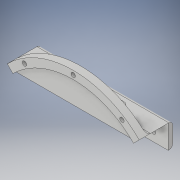
# Autodesk Inventor part: BearingGuard
Saved by Autodesk Inventor 2018 (Build 220112000, 112)
## iProperties
Created: 2019-02-07
Part Number: BearingGuard
Material: Generic
Document SubType Name: Modeling
Designer: anirudh
Density: 1 g/cm^3
Appearance: Default
Author: anirudh
Autodesk Inventor part; units mm, degrees
ref_plane "YZ Plane" through (0, 0, 0) normal (1, 0, 0) x (0, 1, 0)
ref_plane "XZ Plane" through (0, 0, 0) normal (0, 1, 0) x (-1, 0, 0)
ref_plane "XY Plane" through (0, 0, 0) normal (0, 0, 1) x (1, 0, 0)
sketch "Sketch1" plane through (0, 0, 0) normal (0, 0, 1) x (1, 0, 0)
  line L0 (0, 0) -> (101.6, 0)
  arc A0 (101.7181, 101.7181) -> (-0.1181, 101.7181) centre (50.8, 50.8) ccw
  arc A1 (106.4776, 106.4776) -> (-4.8776, 106.4776) centre (50.8, 50.8) ccw
  line L1 (0, 101.6) -> (-4.8776, 106.4776)
  line L2 (0, 101.6) -> (11.1798, 101.6) construction
  line L3 (101.6, 101.6) -> (106.4776, 106.4776)
  constraints: 8 end point, 4 point on circle, 2 centre point, 2 horizontal, 2 point on line, 1 coincident
extrude "Extrusion1" add sketch "Sketch1" along normal blind 2.54
sketch "Sketch2" plane through (0, 0, 0) normal (0, 0, -1) x (-1, 0, 0)
  line L0 (-101.7181, 101.7181) -> (0.1181, 101.7181)
  line L1 (-101.7181, 101.7181) -> (-106.4776, 106.4776) projected
  line L2 (-101.7181, 101.7181) -> (-106.4776, 106.4776)
  line L3 (4.8776, 106.4776) -> (0.1181, 101.7181) projected
  line L4 (0.1181, 101.7181) -> (4.8776, 106.4776)
  arc A0 (4.8776, 106.4776) -> (-106.4776, 106.4776) centre (-50.8, 50.8) ccw projected
  arc A1 (-106.4776, 106.4776) -> (-106.4776, 106.4776) centre (-50.8, 50.8) ccw
  point P0 (0, 0)
  constraints: 6 end point, 2 collinear, 1 horizontal, 4 other
extrude "Extrusion2" add sketch "Sketch2" along normal blind 3.81 contours L1 A0 L3 L0
sketch "Sketch8" plane through (0, 0, 2.54) normal (0, 0, 1) x (1, 0, 0)
  circle A0 centre (9.6434, 113.9463) radius 1.85
  circle A1 centre (50.8, 126.1745) radius 1.85
  circle A2 centre (91.9566, 113.9463) radius 1.85
  point P0 (0, 0)
  dimension "d32" = 3.7
  dimension "d33" = 3.7
  dimension "d34" = 3.7
  constraints: 3 centre point
  measures "d32" diameter of A0
  measures "d33" diameter of A1
  measures "d34" diameter of A2
extrude "Extrusion7" cut sketch "Sketch8" against normal blind 18.0594
sketch "Sketch9" plane through (0, 0, -3.81) normal (0, 0, -1) x (-1, 0, 0)
  line L0 (0.1181, 101.7181) -> (-71.0019, 101.7181)
  line L1 (0.1181, 101.7181) -> (4.8776, 106.4776) projected
  line L2 (0.1181, 101.7181) -> (4.8776, 106.4776)
  line L3 (4.8776, 106.4776) -> (-71.0019, 106.4776)
  arc A0 (4.8776, 106.4776) -> (-106.4776, 106.4776) centre (-50.8, 50.8) ccw projected
  line L4 (-71.0019, 106.4776) -> (4.8776, 106.4776)
  line L5 (-106.4776, 106.4776) -> (-101.7181, 101.7181) projected
  line L6 (-106.4776, 106.4776) -> (-101.7181, 101.7181)
  line L7 (-101.7181, 101.7181) -> (-71.0019, 101.7181)
  line L8 (-101.7181, 101.7181) -> (0.1181, 101.7181) projected
  line L9 (-106.4776, 106.4776) -> (-71.0019, 106.4776)
  point P0 (0, 0)
  dimension "d37" = 71.12
  constraints: 14 end point, 3 collinear, 3 horizontal
  measures "d37" distance of L0.start L0.end
extrude "Extrusion8" add sketch "Sketch9" along normal blind 21.8694 contours L0 L7 L5 L9 L3 L1
sketch "Sketch13" plane through (0, 0, -25.6794) normal (0, 0, -1) x (-1, 0, 0)
  line L0 (-106.4776, 106.4776) -> (-101.7181, 101.7181) projected
  line L1 (4.8776, 106.4776) -> (-106.4776, 106.4776) projected
  line L2 (0, 106.4776) -> (-101.7181, 106.4776)
  line L3 (-101.7181, 106.4776) -> (-101.7181, 86.7181)
  line L4 (-101.7181, 86.7181) -> (0, 86.7181)
  line L5 (0, 86.7181) -> (0, 106.4776)
  point P0 (0, 0)
  constraints: 8 end point, 2 parallel, 1 horizontal, 1 perpendicular, 1 point on line
extrude "Extrusion11" add sketch "Sketch13" along normal blind 3.81 contours L3 L1 L5 L4
sketch "Sketch16" plane through (0, 0, -25.6794) normal (0, 0, -1) x (-1, 0, 0)
  line L0 (4.8776, 106.4776) -> (0.1181, 101.7181) projected
  line L1 (4.8776, 106.4776) -> (0, 106.4776)
  line L2 (-106.4776, 106.4776) -> (4.8776, 106.4776) projected
  line L3 (0, 106.4776) -> (0, 101.7181) projected
  line L4 (0, 106.4776) -> (0, 101.7181)
  line L5 (0, 101.7181) -> (4.8776, 106.4776)
  line L6 (-101.7181, 106.4776) -> (-106.4776, 106.4776) projected
  line L7 (-106.4776, 106.4776) -> (-101.7181, 106.4776)
  line L8 (-106.4776, 106.4776) -> (-101.7181, 101.7181) projected
  line L9 (-101.7181, 106.4776) -> (-101.7181, 101.7181)
  line L10 (-101.7181, 101.7181) -> (-106.4776, 106.4776)
  point P0 (0, 0)
  constraints: 12 end point, 2 collinear, 1 perpendicular, 1 point on line, 1 vertical
extrude "Extrusion13" add sketch "Sketch16" along normal blind 3.81
sketch "Sketch18" plane through (0, 0, -29.4894) normal (0, 0, -1) x (-1, 0, 0)
  line L0 (4.8776, 106.4776) -> (0.1181, 101.7181) projected
  line L1 (-106.4776, 106.4776) -> (4.8776, 106.4776) projected
  line L2 (4.8776, 106.4776) -> (-106.4776, 106.4776)
  line L3 (-101.7181, 101.7181) -> (-106.4776, 106.4776) projected
  line L4 (-106.4776, 106.4776) -> (-101.7181, 101.7181)
  line L5 (-101.7181, 86.7181) -> (-101.7181, 101.7181) projected
  line L6 (-101.7181, 101.7181) -> (-101.7181, 86.7181)
  line L7 (0, 86.7181) -> (-101.7181, 86.7181) projected
  line L8 (-101.7181, 86.7181) -> (0, 86.7181)
  line L9 (0, 86.7181) -> (0, 101.6)
  line L10 (0, 101.6) -> (4.8776, 106.4776)
  point P0 (0, 0)
  constraints: 12 end point, 3 collinear, 3 perpendicular
sketch "Sketch19" plane through (0, 0, -25.6794) normal (0, 0, 1) x (1, 0, 0)
  line L0 (0, 86.7181) -> (101.7181, 86.7181) projected
  line L1 (101.7181, 86.7181) -> (101.7181, 101.7181) projected
  line L2 (0, 86.7181) -> (101.7181, 86.7181)
  line L3 (101.7181, 86.7181) -> (101.7181, 101.7181)
  line L4 (101.7181, 101.7181) -> (0, 101.7181)
  line L5 (0, 101.7181) -> (0, 86.7181)
  point P0 (0, 0)
  constraints: 8 end point, 2 parallel, 1 horizontal, 1 perpendicular
extrude "Extrusion15" add sketch "Sketch19" along normal blind 3.81
extrude "Extrusion16" cut sketch "Sketch18" against normal blind 3.81
sketch "Sketch20" plane through (0, 0, -25.6794) normal (0, 0, -1) x (-1, 0, 0)
  line L0 (0, 101.7181) -> (0, 86.7181) projected
  line L1 (0, 86.7181) -> (-15, 86.7181)
  line L2 (-15, 86.7181) -> (-15, 101.7181)
  line L3 (-15, 101.7181) -> (0, 101.7181)
  line L4 (0, 101.7181) -> (0, 86.7181)
  line L5 (-101.7181, 86.7181) -> (-101.7181, 101.7181) projected
  line L6 (-101.7181, 86.7181) -> (-86.7181, 86.7181)
  line L7 (-86.7181, 86.7181) -> (-86.7181, 101.7181)
  line L8 (-86.7181, 101.7181) -> (-101.7181, 101.7181)
  line L9 (-101.7181, 101.7181) -> (-101.7181, 86.7181)
  circle A0 centre (-94.2181, 94.2181) radius 1.85
  circle A1 centre (-7.5, 94.2181) radius 1.85
  point P0 (0, 0)
  dimension "d89" = 15
  dimension "d90" = 15
  dimension "d91" = 15
  dimension "d92" = 15
  dimension "d93" = 3.7
  dimension "d94" = 3.7
  constraints: 16 end point, 4 parallel, 2 centre point, 2 horizontal, 2 perpendicular
  measures "d89" distance of L2.end L3.end
  measures "d90" distance of L1.end L2.end
  measures "d91" distance of L8.end L7.end
  measures "d92" distance of L7.end L6.end
  measures "d93" diameter of A0
  measures "d94" diameter of A1
extrude "Extrusion17" cut sketch "Sketch20" against normal blind 7.62 contours A0 | A1
sketch "Sketch21" plane through (-4.8776, 106.4776, -3.81) normal (0, 1, 0) x (1, 0, 0)
  line L0 (106.5956, -3.81) -> (106.5956, 18.0594) projected
  circle A0 centre (35.2395, 10.0594) radius 5.35
  circle A1 centre (76.1156, 10.0594) radius 5.35
  point P0 (4.8776, -3.81)
  dimension "d106" = 10.7
  dimension "d107" = 10.7
  constraints: 2 centre point
  measures "d106" diameter of A0
  measures "d107" diameter of A1
extrude "Extrusion19" cut sketch "Sketch21" against normal blind 7.62
sketch "Sketch22" plane through (0, 0, -25.6794) normal (0, 0, -1) x (-1, 0, 0)
  line L0 (0, 101.7181) -> (0, 86.7181) projected
  line L1 (0, 86.7181) -> (-15, 86.7181)
  line L2 (-15, 86.7181) -> (-15, 101.7181)
  line L3 (-15, 101.7181) -> (0, 101.7181)
  line L4 (0, 101.7181) -> (0, 86.7181)
  line L5 (0, 86.7181) -> (-101.7181, 86.7181) projected
  line L6 (-101.7181, 86.7181) -> (-86.7181, 86.7181)
  line L7 (-86.7181, 86.7181) -> (-86.7181, 101.7181)
  line L8 (-86.7181, 101.7181) -> (-101.7181, 101.7181)
  line L9 (-101.7181, 101.7181) -> (-101.7181, 86.7181)
  line L10 (-15, 101.7181) -> (-86.7181, 101.7181)
  line L11 (-86.7181, 101.7181) -> (-86.7181, 86.7181)
  line L12 (-86.7181, 86.7181) -> (-15, 86.7181)
  line L13 (-15, 86.7181) -> (-15, 101.7181)
  arc A0 (-15, 86.7181) -> (-86.7181, 86.7181) centre (-50.859, 4.7434) ccw
  point P0 (0, 0)
  dimension "d114" = 15
  dimension "d115" = 15
  dimension "d116" = 15
  dimension "d117" = 15
  constraints: 24 end point, 6 parallel, 3 horizontal, 3 perpendicular, 2 point on circle, 1 centre point
  measures "d114" distance of L2.end L3.end
  measures "d115" distance of L1.end L2.end
  measures "d116" distance of L8.end L7.end
  measures "d117" distance of L7.end L6.end
extrude "Extrusion20" cut sketch "Sketch22" against normal blind 7.62 contours L5 A0
sketch "Sketch23" plane through (0, 86.7181, -25.6794) normal (-1, 0, 0) x (0, 0, 1)
  line L0 (3.81, 15) -> (3.81, 0) projected
  line L1 (21.8694, 19.7595) -> (0, 19.7595) projected
  line L2 (3.81, 0) -> (0, 0)
  line L3 (0, 0) -> (0, 19.7595)
  line L4 (0, 19.7595) -> (3.81, 19.7595)
  line L5 (3.81, 19.7595) -> (3.81, 0)
  point P0 (25.6794, -86.7181)
  constraints: 8 end point, 2 parallel, 1 horizontal, 1 perpendicular
extrude "Extrusion21" add sketch "Sketch23" along normal blind 4.8768
sketch "Sketch24" plane through (101.7181, 86.7181, -25.6794) normal (1, 0, 0) x (0, 0, -1)
  line L0 (-3.81, 0) -> (-3.81, 19.7587) projected
  line L1 (0, 0) -> (-3.81, 0)
  line L2 (-3.81, 0) -> (-3.81, 19.7587)
  line L3 (-3.81, 19.7587) -> (0, 19.7587)
  line L4 (0, 19.7587) -> (0, 0)
  point P0 (-25.6794, -86.7181)
  constraints: 8 end point, 2 parallel, 1 horizontal, 1 perpendicular
extrude "Extrusion22" add sketch "Sketch24" along normal blind 4.8768
fillet "Fillet11" radius 3.175 5 edges at (50.8, 106.4776, -3.81) (50.8, 106.4776, -25.6794) (50.859, 94.2181, -25.6794) (5.0616, 86.7181, -25.6794) (96.6565, 86.7181, -25.6794)
body "Solid1"
